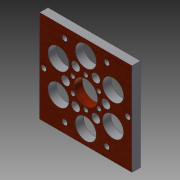
# Autodesk Inventor part: Статор цевков
Saved by Autodesk Inventor 2013 (Build 170138000, 138)
## iProperties
Created: 2014-04-30
Part Number: Статор цевков
Material: Типовые
Document SubType Name: Modeling
Designer: HP1
Density: 1 g/cm^3
Mass: 77.803 g
Surface Area: 295.11 cm^2
Volume: 77.803 cm^3
Author: HP1
Autodesk Inventor part; units mm, degrees
ref_plane "YZ Plane" through (0, 0, 0) normal (1, 0, 0) x (0, 1, 0)
ref_plane "XZ Plane" through (0, 0, 0) normal (0, 1, 0) x (-1, 0, 0)
ref_plane "XY Plane" through (0, 0, 0) normal (0, 0, 1) x (1, 0, 0)
sketch "Эскиз1" plane through (0, 0, 0) normal (0, 1, 0) x (-1, 0, 0)
  circle A0 centre (0, 0) radius 14
  circle A1 centre (0, 0) radius 24 construction
  circle A2 centre (0, 0) radius 55
  circle A3 centre (23.9999, 0) radius 5
  circle A4 centre (12, 20.7845) radius 5
  circle A5 centre (-12, 20.7845) radius 5
  circle A6 centre (-23.9999, 0) radius 5
  circle A7 centre (-12, -20.7845) radius 5
  circle A8 centre (12, -20.7845) radius 5
  line L0 (-54.9999, -55) -> (54.9999, -55)
  line L1 (54.9999, -55) -> (54.9999, 55)
  line L2 (54.9999, 55) -> (-54.9999, 55)
  line L3 (-54.9999, 55) -> (-54.9999, -55)
  line L4 (-54.9999, -55) -> (54.9999, 55) construction
  line L5 (54.9999, -55) -> (-54.9999, 55) construction
  dimension "d0" = 28
  dimension "d1" = 48
  dimension "d2" = 110
  dimension "d3" = 10
  dimension "d6" = 360
  constraints: 12 end point, 9 centre point, 2 midpoint, 2 parallel, 1 perpendicular, 13 other
  measures "d0" diameter of A0
  measures "d1" diameter of A1
  measures "d2" diameter of A2
  measures "d3" diameter of A3
extrude "Выдавливание1" add sketch "Эскиз1" along normal blind 10
sketch "Эскиз2" plane through (0, 10, 0) normal (0, 1, 0) x (1, 0, 0)
  circle A0 centre (0, 0) radius 14 projected
  circle A1 centre (0, 37.5) radius 12.5
  circle A2 centre (-32.476, 18.75) radius 12.5
  circle A3 centre (-32.476, -18.75) radius 12.5
  circle A4 centre (0, -37.5) radius 12.5
  circle A5 centre (32.476, -18.75) radius 12.5
  circle A6 centre (32.476, 18.75) radius 12.5
  dimension "d10" = 25
  dimension "d13" = 360
  dimension "d19" = 37.5
  constraints: 6 centre point, 13 other
  measures "d10" diameter of A1
  measures "d19" distance of A0.centre A1.centre
extrude "Выдавливание2" cut sketch "Эскиз2" against normal blind 10 contours A1 | A2 | A3 | A4 | A5 | A6
sketch "Эскиз3" plane through (0, 10, 0) normal (0, 1, 0) x (1, 0, 0)
  circle A0 centre (0, 0) radius 55 projected
  circle A1 centre (0, 0) radius 14 projected
  circle A2 centre (0, 18) radius 2.5
  circle A3 centre (-15.5885, 9) radius 2.5
  circle A4 centre (-15.5885, -9) radius 2.5
  circle A5 centre (0, -18) radius 2.5
  circle A6 centre (15.5885, -9) radius 2.5
  circle A7 centre (15.5885, 9) radius 2.5
  point P0 (44.976, 18.75)
  point P1 (12.5, 37.5)
  dimension "d20" = 5
  dimension "d22" = 18
  dimension "d25" = 360
  constraints: 6 centre point, 14 other
  measures "d20" diameter of A2
  measures "d22" distance of point (0, 0) A2.centre
extrude "Выдавливание3" cut sketch "Эскиз3" against normal blind 10 contours A2 | A3 | A4 | A5 | A6 | A7
sketch "Эскиз4" plane through (0, 10, 0) normal (0, 1, 0) x (1, 0, 0)
  circle A0 centre (0, 0) radius 14 projected
  circle A1 centre (50, 0) radius 3
  circle A2 centre (25, 43.3013) radius 3
  circle A3 centre (-25, 43.3013) radius 3
  circle A4 centre (-50, 0) radius 3
  circle A5 centre (-25, -43.3013) radius 3
  circle A6 centre (25, -43.3013) radius 3
  dimension "d29" = 6
  dimension "d30" = 50
  dimension "d33" = 360
  constraints: 6 centre point, 13 other
  measures "d29" diameter of A1
  measures "d30" distance of A0.centre A1.centre
extrude "Выдавливание4" cut sketch "Эскиз4" against normal blind 10 contours A1 | A2 | A3 | A4 | A5 | A6
